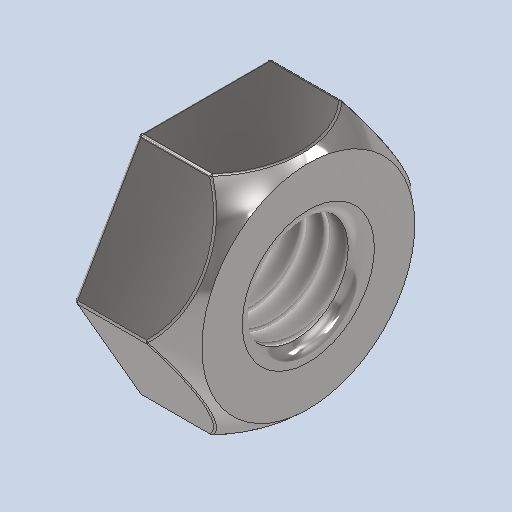
# Autodesk Inventor part: M4_Nut
Saved by Autodesk Inventor 2023 (Build 270158000, 158)
## iProperties
Created: 2020-02-10
Part Number: M4_Nut
Material: 鉄、鋳鉄
Document SubType Name: Modeling
Designer: Hagihara Yuya
Density: 7.15 g/cm^3
Appearance: 鋼 - つや出し
Author: Hagihara Yuya
Autodesk Inventor part; units mm, degrees
ref_plane "YZ Plane" through (0, 0, 0) normal (1, 0, 0) x (0, 1, 0)
ref_plane "XZ Plane" through (0, 0, 0) normal (0, 1, 0) x (-1, 0, 0)
ref_plane "XY Plane" through (0, 0, 0) normal (0, 0, 1) x (1, 0, 0)
sketch "スケッチ1" plane through (0, 0, 0) normal (1, 0, 0) x (0, 1, 0)
  line L0 (0, -3.9837) -> (-3.45, -1.9919)
  line L1 (-3.45, -1.9919) -> (-3.45, 1.9919)
  line L2 (-3.45, 1.9919) -> (0, 3.9837)
  line L3 (0, 3.9837) -> (3.45, 1.9919)
  line L4 (3.45, 1.9919) -> (3.45, -1.9919)
  line L5 (3.45, -1.9919) -> (0, -3.9837)
  line L6 (0, -5.5772) -> (0, 5.5772) projected
  point P0 (0, 0)
  point P1 (0, 0)
  dimension "d0" = 6.9
  constraints: 12 end point, 1 coincident, 1 point on line, 13 other
  measures "d0" distance between parallel lines of L1 L4
extrude "押し出し1" add sketch "スケッチ1" along normal blind 3.2
sketch "スケッチ2" plane through (3.2, 0, 0) normal (1, 0, 0) x (0, 0, -1)
  point P0 (0, 0)
  point P1 (0, 0)
  constraints: 1 coincident
hole "穴1" at (3.2, 0, 0) direction (-1, 0, 0) diameter 3.242 end through all thread size "M4x0.7" class "6H" standard "ISO Metric profile"
sketch "スケッチ5" plane through (0, 0, 0) normal (0, 1, 0) x (-1, 0, 0)
  circle A0 centre (-0.0681, 0) radius 4.5183
  line L0 (5.6865, 0) -> (-7.0039, 0) projected
  line L1 (0, 1.9919) -> (0, 3.9837) projected
  line L2 (0, 3.9837) -> (-3.2, 3.9837) projected
  line L3 (-3.2, -1.9919) -> (-3.2, -3.9837) projected
  circle A1 centre (-0.0681, 0) radius 5.0675
  point P0 (0, 0)
  point P1 (-2.2, 3.9837)
  point P2 (-3.1, 3.35)
  point P3 (-5.1355, 0)
  point P4 (-4.5864, 0)
  point P5 (4.4503, 0)
  point P6 (4.9994, 0)
  dimension "d14" = 2.2
  dimension "d15" = 3.35
  dimension "d16" = 3.1
  constraints: 2 point on circle, 2 point on line, 1 centre point, 1 coincident, 3 other
  measures "d14" distance of L1.end A0.start
  measures "d15" distance from line of L0 A0.end
  measures "d16" distance from line of L1 A0.end
revolve "回転1" cut sketch "スケッチ5" angle 360 about axis through (-10, 0, 0) along (1, 0, 0) contours A0 L2 A1 L0 | A0 L0 A1 L2
fillet "フィレット1" radius 0.1 12 edges at (1.1, 0, 3.9837) (1.1, -3.45, 1.9919) (1.1, -3.45, -1.9919) (1.1, 0, -3.9837) (1.1, 3.45, -1.9919) (1.1, 3.45, 1.9919) (0, 3.45, 0) (0, 1.725, 2.9878) (0, 1.725, -2.9878) (0, -1.725, -2.9878) (0, -3.45, 0) (0, -1.725, 2.9878)
fillet "フィレット2" radius 0.4 2 edges at (3.2, 0, 1.621) (0, 0, 1.621)
fillet "フィレット3" radius 0.1 13 edges at (2.2348, -0.0259, 3.9648) (2.2287, -3.4366, 1.9841) (2.2287, 3.4366, 1.9841) (2.2348, 0.0259, 3.9648) (2.9857, 1.725, 2.9878) (2.9857, 3.45, 0) (2.2287, 3.4366, -1.9841) (2.9857, 1.725, -2.9878) (2.2287, 0, -3.9682) (2.9857, -1.725, -2.9878) (2.2287, -3.4366, -1.9841) (2.9857, -3.45, 0) (2.9857, -1.725, 2.9878)
